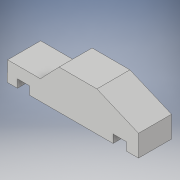
# Autodesk Inventor part: idek
Saved by Autodesk Inventor 2017 (Build 210142000, 142)
## iProperties
Created: 2018-09-10
Part Number: idek
Material: Generic
Document SubType Name: Modeling
Designer: qthuynh
Density: 1 g/cm^3
Appearance: Default
Author: qthuynh
Autodesk Inventor part; units mm, degrees
ref_plane "YZ Plane" through (0, 0, 0) normal (1, 0, 0) x (0, 1, 0)
ref_plane "XZ Plane" through (0, 0, 0) normal (0, 1, 0) x (-1, 0, 0)
ref_plane "XY Plane" through (0, 0, 0) normal (0, 0, 1) x (1, 0, 0)
sketch "Sketch1" plane through (0, 0, 0) normal (0, 0, 1) x (1, 0, 0)
  line L0 (5.5548, -13.9824) -> (-146.8452, -13.9824)
  line L1 (-146.8452, -13.9824) -> (-146.8452, 138.4176)
  line L2 (-146.8452, 138.4176) -> (5.5548, 138.4176)
  line L3 (5.5548, 138.4176) -> (5.5548, -13.9824)
  point P0 (0, 0)
  dimension "d0" = 152.4
  dimension "d1" = 152.4
  constraints: 8 end point, 2 parallel, 1 horizontal, 1 perpendicular
  measures "d0" distance of L1.end L2.end
  measures "d1" distance of L0.end L1.end
extrude "Extrusion1" add sketch "Sketch1" along normal blind 152.4
sketch "Sketch2" plane through (0, 0, 152.4) normal (0, 0, 1) x (1, 0, 0)
  line L0 (-7.9985, 123.7101) -> (68.2015, 123.7101)
  line L1 (68.2015, 123.7101) -> (68.2015, 199.9101)
  line L2 (68.2015, 199.9101) -> (-7.9985, 199.9101)
  line L3 (-7.9985, 199.9101) -> (-7.9985, 123.7101)
  point P0 (0, 0)
  dimension "d4" = 76.2
  dimension "d5" = 76.2
  constraints: 8 end point, 2 parallel, 1 horizontal, 1 perpendicular
  measures "d4" distance of L2.end L1.end
  measures "d5" distance of L1.end L0.end
extrude "Extrusion2" add sketch "Sketch2" along normal blind 76.2
sketch "Sketch3" plane through (0, 0, 152.4) normal (0, 0, 1) x (1, 0, 0)
  line L0 (-139.924, 111.3869) -> (-133.2191, 100.298)
  line L1 (-133.2191, 100.298) -> (-125.2248, 109.0659)
  line L2 (-125.2248, 109.0659) -> (-133.2191, 100.298)
  line L3 (-133.2191, 84.3093) -> (-133.2191, 100.298)
  line L4 (-115.6832, 84.3093) -> (-115.6832, 109.0659)
  line L5 (-115.6832, 109.0659) -> (-102.5313, 109.0659)
  line L6 (-102.5313, 109.0659) -> (-115.6832, 109.0659)
  line L7 (-115.6832, 96.6876) -> (-109.1072, 96.6876)
  line L8 (-109.1072, 96.6876) -> (-115.6832, 96.6876)
  line L9 (-115.6832, 84.3093) -> (-102.5313, 84.3093)
  line L10 (-93.2475, 84.3093) -> (-93.2475, 109.0659)
  line L11 (-93.2475, 109.0659) -> (-80.8692, 109.0659)
  line L12 (-80.8692, 109.0659) -> (-93.2475, 109.0659)
  line L13 (-93.2475, 96.6876) -> (-87.0584, 96.6876)
  line L14 (-87.0584, 96.6876) -> (-93.2475, 96.6876)
  line L15 (-93.2475, 85.5987) -> (-93.2475, 84.3093)
  line L16 (-93.2475, 84.3093) -> (-80.8692, 84.3093)
  line L17 (-80.8692, 84.3093) -> (-93.2475, 84.3093)
  line L18 (-70.8119, 109.0659) -> (-50.6971, 109.0659)
  line L19 (-50.6971, 109.0659) -> (-60.7545, 109.0659)
  line L20 (-60.7545, 84.3093) -> (-60.7545, 109.0659)
  point P0 (0, 0)
  constraints: 42 end point, 6 collinear, 5 horizontal, 4 perpendicular, 3 midpoint, 2 vertical, 1 point on line
sketch "Sketch4" plane through (0, 0, 152.4) normal (0, 0, 1) x (1, 0, 0)
  circle A0 centre (105.4068, -100.1365) radius 100.0904
  line L0 (328.5178, -219.5975) -> (520.0068, -22.8381)
  point P0 (0, 0)
  constraints: 2 end point, 1 centre point
revolve "Revolution1" add sketch "Sketch4" angle 360 about axis through (328.5178, -219.5975, 152.4) along (0.6974, 0.7166, 0)
sketch "Sketch5" plane through (0, 0, 152.4) normal (0, 0, 1) x (1, 0, 0)
  point P0 (0, 0)
sketch "Sketch6" plane through (0, 0, 152.4) normal (0, 0, 1) x (1, 0, 0)
  line L0 (-650.7364, 19.5577) -> (-1158.7364, 19.5577)
  line L1 (-1158.7364, 19.5577) -> (-1158.7364, 527.5577)
  line L2 (-1158.7364, 527.5577) -> (-650.7364, 527.5577)
  line L3 (-650.7364, 527.5577) -> (-650.7364, 19.5577)
  line L4 (-578.6879, 19.5577) -> (-578.6879, 416.9476)
  dimension "d9" = 508
  dimension "d10" = 508
  constraints: 10 end point, 2 parallel, 1 horizontal, 1 perpendicular, 1 vertical
  measures "d9" distance of L1.end L2.end
  measures "d10" distance of L0.end L1.end
revolve "Revolution2" add sketch "Sketch6" angle 360 about axis through (-578.6879, 19.5577, 152.4) along (0, 1, 0)
sketch "Sketch7" plane through (0, 0, 152.4) normal (0, 0, 1) x (1, 0, 0)
  arc A0 (748.0487, 663.7921) -> (743.2615, 668.3592) centre (483.9842, 391.7968) ccw construction
  arc A1 (973.1233, 895.6265) -> (964.2557, 904.0864) centre (483.9842, 391.7968) ccw
  arc A2 (522.9741, 431.9577) -> (522.2672, 432.632) centre (483.9842, 391.7968) ccw
  arc A3 (522.9741, 431.9577) -> (973.1233, 895.6265) centre (748.0487, 663.7921) ccw
  arc A4 (964.2557, 904.0864) -> (522.2672, 432.632) centre (743.2615, 668.3592) ccw
  line L0 (483.9842, 391.7968) -> (748.0487, 663.7921) construction
  line L1 (483.9842, 391.7968) -> (743.2615, 668.3592) construction
  line L2 (1155.2242, 328.4179) -> (1137.9391, 904.0864)
  point P0 (0, 0)
  dimension "d12" = 1
  constraints: 10 point on circle, 6 end point, 5 centre point, 4 tangent
  measures "d12" angle of L0 L1
revolve "Revolution3" add sketch "Sketch7" angle 360 about axis through (1155.2242, 328.4179, 152.4) along (-0.03, 0.9995, 0)
sketch "Sketch8" plane through (0, 0, 152.4) normal (0, 0, 1) x (1, 0, 0)
  line L0 (-1944.3216, 913.6511) -> (-1750.7896, 1350.2233)
  line L1 (-1750.7896, 1350.2233) -> (-1080.1787, 1386.2292)
  line L2 (-1080.1787, 1386.2292) -> (-1061.8477, 1044.816)
  line L3 (-1061.8477, 1044.816) -> (-121.5201, 1044.816)
  line L4 (-121.5201, 1044.816) -> (-229.1827, 801.9493)
  line L5 (-229.1827, 801.9493) -> (-836.8804, 769.3213)
  line L6 (-836.8804, 769.3213) -> (-1701.2814, 923.3827)
  line L7 (-1701.2814, 923.3827) -> (-1503.2486, 504.0833)
  line L8 (-1503.2486, 504.0833) -> (-1269.0809, 8.2745)
  line L9 (-1269.0809, 8.2745) -> (-1813.8, 144.0238)
  line L10 (-1813.8, 144.0238) -> (-1944.3216, 713.733)
  line L11 (-1944.3216, 713.733) -> (-2502.4139, 713.733)
  line L12 (-2502.4139, 713.733) -> (-2695.9459, 1215.5226)
  line L13 (-2695.9459, 1215.5226) -> (-1944.3216, 913.6511)
  point P0 (0, 0)
  constraints: 28 end point, 2 parallel, 2 perpendicular, 1 horizontal, 1 point on line
extrude "Extrusion3" add sketch "Sketch8" along normal blind 1270
sketch "Sketch9" plane through (0, 0, 152.4) normal (0, 0, 1) x (1, 0, 0)
  line L0 (5344.3125, 12228.9393) -> (15395.8429, 22708.1943)
  line L1 (15395.8429, 22708.1943) -> (35766.2316, 22708.1943)
  line L2 (35766.2316, 22708.1943) -> (15395.8429, 22708.1943)
  line L3 (5344.3125, 12228.9393) -> (-12299.3312, 12228.9393)
  line L4 (-12299.3312, 12228.9393) -> (-12566.6592, 1642.7531)
  line L5 (-12566.6592, 1642.7531) -> (-7008.0102, 1642.7531)
  line L6 (-7008.0102, 1642.7531) -> (-7008.0102, 6026.9312)
  line L7 (-7008.0102, 6026.9312) -> (-604.5524, 6026.9312)
  line L8 (-604.5524, 6026.9312) -> (-604.5524, 1642.7531)
  line L9 (-604.5524, 1642.7531) -> (44481.1223, 1642.7531)
  line L10 (44481.1223, 1642.7531) -> (44481.1223, 6026.9312)
  line L11 (44481.1223, 6026.9312) -> (51769.4184, 6026.9312)
  line L12 (51769.4184, 6026.9312) -> (51769.4184, 1642.7531)
  line L13 (51769.4184, 1642.7531) -> (58167.7319, 1642.7531)
  line L14 (58167.7319, 1642.7531) -> (58167.7319, 13211.0547)
  line L15 (58167.7319, 13211.0547) -> (48125.2703, 17468.5668)
  line L16 (48125.2703, 17468.5668) -> (35766.2316, 22708.1943)
  point P0 (0, 0)
  constraints: 34 end point, 7 perpendicular, 3 horizontal, 2 collinear, 2 point on line, 1 parallel, 1 vertical
extrude "Extrusion4" add sketch "Sketch9" along normal blind 17780
body "Solid1"
